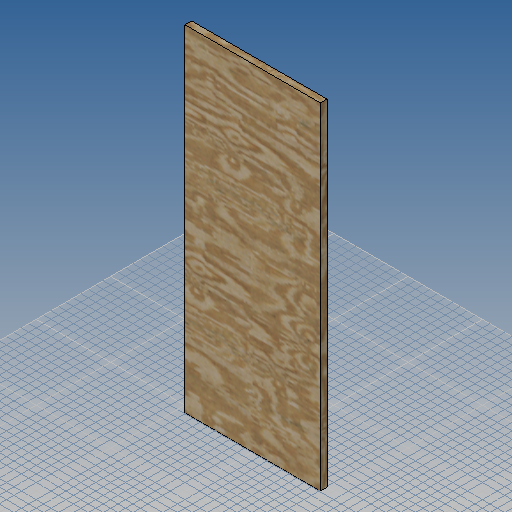
# Autodesk Inventor part: Korpus_Rücken
Saved by Autodesk Inventor 2019 (Build 230136000, 136)
## iProperties
Created: 2020-08-02
Part Number: Korpus_Rücken
Material: Generisch
Document SubType Name: Modeling
Designer: Stefan
Mass: 5923.01 g
Surface Area: 7037.6 cm^2
Volume: 5923.01 cm^3
Density: 1 g/cm^3
Appearance: Sperrholz - verwittert
Author: Stefan
Autodesk Inventor part; units mm, degrees
ref_plane "YZ Plane" through (0, 0, 0) normal (1, 0, 0) x (0, 1, 0)
ref_plane "XZ Plane" through (0, 0, 0) normal (0, 1, 0) x (-1, 0, 0)
ref_plane "XY Plane" through (0, 0, 0) normal (0, 0, 1) x (1, 0, 0)
sketch "Skizze1" plane through (0, 0, 0) normal (0, 0, 1) x (1, 0, 0)
  line L0 (-182, -452) -> (182, -452)
  line L1 (182, -452) -> (182, 452)
  line L2 (182, 452) -> (-182, 452)
  line L3 (-182, 452) -> (-182, -452)
  line L4 (-182, -452) -> (182, 452) construction
  line L5 (182, -452) -> (-182, 452) construction
  point P0 (0, 0)
  dimension "d0" = 904
  dimension "d1" = 364
  constraints: 12 end point, 2 midpoint, 2 parallel, 1 horizontal, 1 perpendicular
  measures "d0" distance of L2.end L0.start
  measures "d1" distance of L1.end L2.end
extrude "Extrusion1" add sketch "Skizze1" along normal blind 18
equation "\"d0\" = case_height - 2 * case_thickness"
equation "\"d1\" = case_width - 2 * case_thickness"
equation "\"d2\" = case_thickness"
equation "\"kg_thickness\" = 4.9"
equation "\"ht_thickness\" = 1.9"
equation "\"case_thickness\" = 18"
equation "\"inner_thickness\" = 15"
equation "\"gap_fit\" = 0.1"
equation "\"gap_slide\" = 0.2"
equation "\"gap_air\" = 1"
equation "\"bore_diameter\" = 73"
equation "\"mdf_thickness\" = 6"
equation "\"tape_width\" = 15"
equation "\"tape_thickness\" = 3"
equation "\"inner_depth\" = 255"
equation "\"case_height\" = 940"
equation "\"case_width\" = 400"
